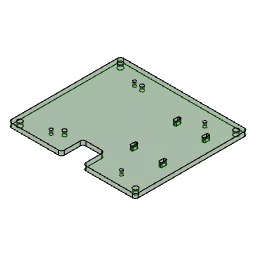
Support_raspberry_KOSMOS3-0 (Autodesk Fusion 360 design; units mm, degrees)
Autodesk Fusion 360 part; units mm, degrees
note: some values were not read from the file. Set by a fixed rule: which sketch regions a step uses.
sketch "Esquisse1" plane through (0, 0, 0) normal (0, 0, 1) x (1, 0, 0)
  line L0 (88.4, 2) -> (88.4, 76)
  line L1 (86.4, 78) -> (2, 78)
  line L2 (0, 76) -> (0, 2)
  circle A0 centre (3.9, 4) radius 1.75
  circle A1 centre (3.9, 74) radius 1.75
  circle A2 centre (84.5, 74) radius 1.75
  circle A3 centre (84.5, 4) radius 1.75
  arc A4 (0, 2) -> (2, 0) centre (2, 2) ccw
  arc A5 (2, 78) -> (0, 76) centre (2, 76) ccw
  arc A6 (88.4, 76) -> (86.4, 78) centre (86.4, 76) ccw
  arc A7 (86.4, 0) -> (88.4, 2) centre (86.4, 2) ccw
  circle A8 centre (19.7, 10) radius 1.05
  circle A9 centre (68.7, 10) radius 1.05
  circle A10 centre (19.7, 68) radius 1.05
  circle A11 centre (68.7, 68) radius 1.05
  line L3 (51.9, 2) -> (51.9, 13)
  line L4 (49.9, 15) -> (38.9, 15)
  line L5 (36.9, 13) -> (36.9, 2)
  line L6 (34.9, 0) -> (2, 0)
  line L7 (86.4, 0) -> (53.9, 0)
  arc A12 (34.9, 0) -> (36.9, 2) centre (34.9, 2) ccw
  arc A13 (51.9, 2) -> (53.9, 0) centre (53.9, 2) ccw
  arc A14 (51.9, 13) -> (49.9, 15) centre (49.9, 13) ccw
  arc A15 (38.9, 15) -> (36.9, 13) centre (38.9, 13) ccw
  circle A16 centre (58.4, 28) radius 1.05
  circle A17 centre (25, 68) radius 1.3
  circle A18 centre (25, 14) radius 1.3
  line L8 (57.9, 28) -> (56.9, 28)
  line L9 (56.4, 28.5) -> (56.4, 31.5)
  line L10 (56.9, 32) -> (57.9, 32)
  line L11 (58.4, 31.5) -> (58.4, 28.5)
  arc A19 (56.4, 28.5) -> (56.9, 28) centre (56.9, 28.5) ccw
  arc A20 (56.9, 32) -> (56.4, 31.5) centre (56.9, 31.5) ccw
  arc A21 (58.4, 31.5) -> (57.9, 32) centre (57.9, 31.5) ccw
  arc A22 (57.9, 28) -> (58.4, 28.5) centre (57.9, 28.5) ccw
  line L12 (77.9, 28) -> (76.9, 28)
  arc A23 (77.9, 28) -> (78.4, 28.5) centre (77.9, 28.5) ccw
  line L13 (78.4, 31.5) -> (78.4, 28.5)
  line L14 (76.4, 28.5) -> (76.4, 31.5)
  arc A24 (76.4, 28.5) -> (76.9, 28) centre (76.9, 28.5) ccw
  line L15 (76.9, 32) -> (77.9, 32)
  arc A25 (78.4, 31.5) -> (77.9, 32) centre (77.9, 31.5) ccw
  arc A26 (76.9, 32) -> (76.4, 31.5) centre (76.9, 31.5) ccw
  line L16 (57.9, 58) -> (56.9, 58)
  arc A27 (57.9, 58) -> (58.4, 58.5) centre (57.9, 58.5) ccw
  line L17 (58.4, 61.5) -> (58.4, 58.5)
  line L18 (56.4, 58.5) -> (56.4, 61.5)
  arc A28 (56.4, 58.5) -> (56.9, 58) centre (56.9, 58.5) ccw
  line L19 (56.9, 62) -> (57.9, 62)
  arc A29 (58.4, 61.5) -> (57.9, 62) centre (57.9, 61.5) ccw
  arc A30 (56.9, 62) -> (56.4, 61.5) centre (56.9, 61.5) ccw
  line L20 (77.9, 58) -> (76.9, 58)
  arc A31 (77.9, 58) -> (78.4, 58.5) centre (77.9, 58.5) ccw
  line L21 (78.4, 61.5) -> (78.4, 58.5)
  line L22 (76.4, 58.5) -> (76.4, 61.5)
  arc A32 (76.4, 58.5) -> (76.9, 58) centre (76.9, 58.5) ccw
  line L23 (76.9, 62) -> (77.9, 62)
  arc A33 (78.4, 61.5) -> (77.9, 62) centre (77.9, 61.5) ccw
  arc A34 (76.9, 62) -> (76.4, 61.5) centre (76.9, 61.5) ccw
  point P0 (88.4, 0)
  point P1 (0, 78)
  point P2 (36.9, 0)
  point P3 (36.9, 15)
  point P4 (58.4, 28)
  point P5 (56.4, 28)
  point P6 (58.4, 32)
  dimension "d1" = 78
  dimension "d2" = 88.4
  dimension "d3" = 3.5
  dimension "d4" = 3.9
  dimension "d6" = 3.5
  dimension "d8" = 4
  dimension "d9" = 3.5
  dimension "d10" = 4
  dimension "d11" = 3.9
  dimension "d12" = 3.5
  dimension "d13" = 3.9
  dimension "d15" = 2
  dimension "d16" = 2
  dimension "d17" = 2
  dimension "d18" = 2
  dimension "d21" = 2.1
  dimension "d24" = 49
  dimension "d25" = 58
  dimension "d28" = 19.7
  dimension "d30" = 15
  dimension "d31" = 36.9
  dimension "d33" = 2
  dimension "d34" = 2
  dimension "d35" = 2
  dimension "d36" = 2
  dimension "d37" = 15
  dimension "d41" = 2.1
  dimension "d44" = 20
  dimension "d45" = 30
  dimension "d46" = 30
  dimension "d47" = 50
  dimension "d48" = 2.6
  dimension "d51" = 0
  dimension "d52" = -54
  dimension "d53" = 10
  dimension "d54" = 25
  dimension "d55" = 2
  dimension "d56" = 4
  dimension "d57" = 0.5
  constraint vertical L0
  constraint horizontal L1
  constraint vertical L2
  constraint coincident origin L2
  constraint tangent L2 A4
  constraint coincident P1 L2
  constraint coincident P1 L1
  constraint tangent L2 A5
  constraint tangent L1 A5
  constraint tangent L1 A6
  constraint tangent L0 A6
  constraint coincident P0 L0
  constraint tangent L0 A7
  constraint vertical L3
  constraint horizontal L4
  constraint vertical L5
  constraint tangent A4 L6
  constraint tangent A7 L7
  constraint coincident P2 L5
  constraint coincident P2 L6
  constraint tangent L5 A12
  constraint tangent L6 A12
  constraint tangent L3 A13
  constraint tangent L7 A13
  constraint tangent L3 A14
  constraint tangent L4 A14
  constraint coincident P3 L4
  constraint coincident P3 L5
  constraint tangent L4 A15
  constraint tangent L5 A15
  constraint horizontal L8
  constraint vertical L9
  constraint horizontal L10
  constraint vertical L11
  constraint coincident P4 A16.centre
  constraint coincident P5 L8
  constraint coincident P5 L9
  constraint tangent L8 A19
  constraint tangent L9 A19
  constraint tangent L9 A20
  constraint tangent L10 A20
  constraint equal A19 A20
  constraint coincident P6 L10
  constraint coincident P6 L11
  constraint tangent L10 A21
  constraint tangent L11 A21
  constraint equal A19 A21
  constraint coincident P4 L8
  constraint coincident P4 L11
  constraint tangent L8 A22
  constraint tangent L11 A22
  constraint equal A19 A22
  measures "d1" distance of origin P1
  measures "d2" distance of origin P0
  measures "d3" diameter of A0
  measures "d4" distance of L2 A0.centre
  measures "d6" diameter of A1
  measures "d8" distance of L1 A1.centre
  measures "d9" diameter of A2
  measures "d10" distance of L1 A2.centre
  measures "d11" distance of L0 A2.centre
  measures "d12" diameter of A3
  measures "d13" distance of L0 A3.centre
  measures "d15" radius of A4
  measures "d16" radius of A5
  measures "d17" radius of A6
  measures "d18" radius of A7
  measures "d21" diameter of A8
  measures "d28" distance of L2 A8.centre
  measures "d30" distance of P2 P3
  measures "d31" distance of L2 L5
  measures "d33" radius of A12
  measures "d34" radius of A13
  measures "d35" radius of A14
  measures "d36" radius of A15
  measures "d37" distance of L3 L5
  measures "d41" diameter of A16
  measures "d46" distance of L0 P4
  measures "d47" distance of L1 P4
  measures "d48" diameter of A17
  measures "d53" distance of L1 A17.centre
  measures "d54" distance of L2 A17.centre
  measures "d55" distance of P4 P5
  measures "d56" distance of P4 P6
  measures "d57" radius of A19
extrude "Extrusion1" add sketch "Esquisse1" along normal blind 3 contours L0 L1 L2 A4 A5 A6 A7 L3 L4 L5 L6 L7 A12 A13 A14 A15 | A16 L8 L11 A22 picked at (58.8173, 27.529)
